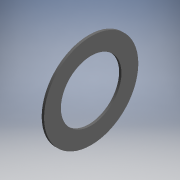
# Autodesk Inventor part: 684AZZ Shield2
Saved by Autodesk Inventor 2017.3 (Build 213256000, 256)
## iProperties
Part Number: 684AZZ Shield2
Material: Generic
Catalog Web Link: www.cadenas.de
Description: shielde_type_zz_zzs_S2-
Vendor: NSK_RB
Document SubType Name: Modeling
Designer: partserver
Manufacturer: NSK_RB
Mass: 0.00603433 g
Surface Area: 0.689088 cm^2
Volume: 0.00603433 cm^3
Density: 1 g/cm^3
Appearance: PSOLRGB-128-128-128
Category: PARTsolutions
Company: NSK_RB
Title: 684AZZ Shield2
Author: Cadenas PARTsolutions
PSOL_IDENT_0: {$CADENAS_DATA\23d-libs\nsk_rb\roller_bearings\deep_groove_bb\exstra_small_miniatur_bb\metric_design
PSOL_IDENT_1: \shielded_type_zz_zzs_s2.prj},185 {VTYP=3D},{NB=684AZZ Shield2},{LINA=684AZZ Shield2},{NN=shielde_ty
PSOL_IDENT_2: pe_zz_zzs_S2},{DATE=30.03.2022 01:55:07},{GEOMDATE=04.01.2008 00:00:00},{VERSION=},{LINEID=220},{WBV
PSOL_IDENT_3: AR=},{WBNUMERIC=}  {NB=684AZZ Shield2},{LINA=684AZZ Shield2},{KT=DUMMY},{IDNR=},{STAN=Standard},{ORD
PSOL_IDENT_4: ER=684AZZ},{SD=4.0},{X=4.0},{DI1=5.20},{DI2=5.20},{SDE1=7.50},{SDE2=8.10},{D=9},{DD=9},{B=0.0},{B1=4
PSOL_IDENT_5: .0},{R=0.00},{R1=0.15},{CR1=640},{COR1=225},{CR2=65},{COR2=23.0},{LG=53000},{LO=63000},{DA=0.0},{DB=
PSOL_IDENT_6: 5.2},{DA1=0.0},{DB1=8.1},{RA=0.00},{RB=0.10},{MASS=1.01},{SC=1}
NB: 684AZZ Shield2
NN: shielde_type_zz_zzs_S2
NBSYN: $ORDER. Shield2
LINA: 684AZZ Shield2
CATALOG: NSK Rolling Bearing
STAN: Standard
ORDER: 684AZZ
SD: 4
X: 4
DI1: 5.2
DI2: 5.2
SDE1: 7.5
SDE2: 8.1
D: 9
DD: 9
B: 0
B1: 4
R: 0
R1: 0.15
CR1: 640
COR1: 225
CR2: 65
COR2: 23
LG: 53000
LO: 63000
DA: 0
DB: 5.2
DA1: 0
DB1: 8.1
RA: 0
RB: 0.1
MASS: 1.01
SC: 1
SUPPLIER: NSK_RB
ARTICLENO: 684AZZ Shield2
BOMINFO: 684AZZ Shield2
CREATOR: CADENAS GmbH
Autodesk Inventor part; units mm, degrees
sketch "Sketch_1" plane through (0, 0, 0) normal (0, 0, 1) x (1, 0, 0)
  line L0 (3.9336, 0) -> (3.7344, 0)
  line L1 (3.7344, 2.6) -> (3.9336, 2.6)
  line L2 (3.9336, 2.6) -> (3.9336, 4.05)
  line L3 (3.9336, 4.05) -> (3.7344, 4.05)
  line L4 (3.7344, 4.05) -> (3.7344, 2.6)
  constraints: 10 end point
revolve "Revolution1" add sketch "Sketch_1" angle 360 about axis through (3.9336, 0, 0) along (1, 0, 0)
ref_plane "ip_st_s2_XY" through (3.7344, 0, 0) normal (1, 0, 0) x (0, 0, -1)
ref_plane "ip_st_s2_YZ" through (3.7344, 0, 0) normal (0, 0, -1) x (0, 1, 0)
ref_plane "ip_st_s2_ZX" through (3.7344, 0, 0) normal (0, 1, 0) x (1, 0, 0)
body "Solid1"
